# Autodesk Inventor part: SFE_LOGO_NAME_FLAME_1_INCH
Saved by Autodesk Inventor 2016 SP1 (Build 200210100, 210)
## iProperties
Created: 2015-11-19
Part Number: SFE_LOGO_NAME_FLAME_1_INCH
Material: Generic
Document SubType Name: Modeling
Designer: PhillipD
Density: 1 g/cm^3
Appearance: SFE_LOGO_NAME_FLAME__1, SFE_LOGO_NAME_FLAME_1_INCH
Author: PhillipD
Autodesk Inventor part; units mm, degrees
ref_plane "YZ Plane" through (0, 0, 0) normal (1, 0, 0) x (0, 1, 0)
ref_plane "XZ Plane" through (0, 0, 0) normal (0, 1, 0) x (-1, 0, 0)
ref_plane "XY Plane" through (0, 0, 0) normal (0, 0, 1) x (1, 0, 0)
sketch "SFE_LOGO_NAME_FLAME__1, SFE_LOGO_NAME_FLAME_1_INCH_65" plane through (0, 0, 0) normal (0, 0, 1) x (1, 0, 0)
  line L0 (0, 5.19) -> (11.33, 5.19)
  line L1 (11.33, 5.19) -> (11.33, 0)
  line L2 (11.33, 0) -> (0, 0)
  line L3 (0, 0) -> (0, 5.19)
  constraints: 8 end point
extrude "Extrusion1" add sketch "SFE_LOGO_NAME_FLAME__1, SFE_LOGO_NAME_FLAME_1_INCH_65" along normal blind 1
body "Solid1"
